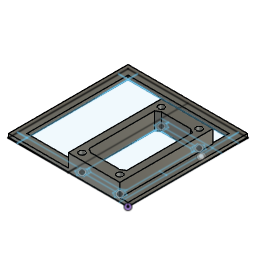
Redstone ESP 8266 Bracket v4 (Autodesk Fusion 360 design; units mm, degrees)
Autodesk Fusion 360 part; units mm, degrees
note: some values were not read from the file. Set by a fixed rule: which sketch regions a step uses.
sketch "Sketch1" plane through (0, 0, 0) normal (0, 0, 1) x (1, 0, 0)
  line L0 (0, 0) -> (-65, 0)
  line L1 (-65, 0) -> (-65, 65)
  line L2 (-65, 65) -> (0, 65)
  line L3 (0, 65) -> (0, 0)
  line L4 (-32.5, 65) -> (-32.5, 0)
  line L5 (-28.75, 1) -> (-26.3684, 2.375)
  line L6 (-26.3684, 2.375) -> (-26.3684, 5.125)
  line L7 (-26.3684, 5.125) -> (-28.75, 6.5)
  line L8 (-28.75, 6.5) -> (-31.1316, 5.125)
  line L9 (-31.1316, 5.125) -> (-31.1316, 2.375)
  line L10 (-31.1316, 2.375) -> (-28.75, 1)
  line L11 (-28.75, 44.19) -> (-26.3684, 45.565)
  line L12 (-26.3684, 45.565) -> (-26.3684, 48.315)
  line L13 (-26.3684, 48.315) -> (-28.75, 49.69)
  line L14 (-28.75, 49.69) -> (-31.1316, 48.315)
  line L15 (-31.1316, 48.315) -> (-31.1316, 45.565)
  line L16 (-31.1316, 45.565) -> (-28.75, 44.19)
  line L17 (-28.75, 49.69) -> (-28.75, 50.69)
  line L18 (-28.75, 50.69) -> (-32.5, 50.69)
  line L19 (-28.75, 50.69) -> (0, 50.69)
  line L20 (-65, 0) -> (-60, 0)
  line L21 (-60, 0) -> (-60, 5)
  line L22 (-60, 5) -> (-65, 5)
  line L23 (-65, 5) -> (-65, 0)
  line L24 (-65, 65) -> (-60, 65)
  line L25 (-60, 65) -> (-60, 60)
  line L26 (-60, 60) -> (-65, 60)
  line L27 (-65, 60) -> (-65, 65)
  line L28 (0, 65) -> (-5, 65)
  line L29 (-5, 65) -> (-5, 60)
  line L30 (-5, 60) -> (0, 60)
  line L31 (0, 60) -> (0, 65)
  line L32 (-5, 60) -> (-60, 60)
  line L33 (-60, 60) -> (-60, 65)
  line L34 (-60, 65) -> (-5, 65)
  line L35 (-5, 65) -> (-5, 60)
  line L36 (-60, 60) -> (-65, 60)
  line L37 (-65, 60) -> (-65, 5)
  line L38 (-65, 5) -> (-60, 5)
  line L39 (-60, 5) -> (-60, 60)
  line L40 (-60, 0) -> (-32.5, 0)
  line L41 (-32.5, 0) -> (-32.5, 5)
  line L42 (-32.5, 5) -> (-60, 5)
  line L43 (-60, 5) -> (-60, 0)
  line L44 (-28.75, 6.5) -> (-28.75, 7.5)
  line L45 (-28.75, 7.5) -> (-26.3684, 6.125)
  line L46 (-28.75, 44.19) -> (-28.75, 43.19)
  line L47 (-3.75, 44.19) -> (-3.75, 43.19)
  line L48 (-26.3684, 44.565) -> (-28.75, 43.19)
  line L49 (-28.75, 7.5) -> (-28.75, 43.19)
  circle A0 centre (-28.75, 46.94) radius 1.65
  circle A1 centre (-28.75, 3.75) radius 1.65
  line L50 (-5, 60) -> (-5, 50.69)
  line L51 (-28.75, 46.94) -> (-8.2, 46.94)
  circle A2 centre (-8.2, 46.94) radius 1.65
  line L52 (-28.75, 3.75) -> (-8.2, 3.75)
  circle A3 centre (-8.2, 3.75) radius 1.65
  line L53 (-8.2, 1) -> (-5.8184, 2.375)
  line L54 (-5.8184, 2.375) -> (-5.8184, 5.125)
  line L55 (-5.8184, 5.125) -> (-8.2, 6.5)
  line L56 (-8.2, 6.5) -> (-10.5816, 5.125)
  line L57 (-10.5816, 5.125) -> (-10.5816, 2.375)
  line L58 (-10.5816, 2.375) -> (-8.2, 1)
  line L59 (-8.2, 44.19) -> (-5.8184, 45.565)
  line L60 (-5.8184, 45.565) -> (-5.8184, 48.315)
  line L61 (-5.8184, 48.315) -> (-8.2, 49.69)
  line L62 (-8.2, 49.69) -> (-10.5816, 48.315)
  line L63 (-10.5816, 48.315) -> (-10.5816, 45.565)
  line L64 (-10.5816, 45.565) -> (-8.2, 44.19)
  line L65 (-8.2, 44.19) -> (-8.2, 43.19)
  line L66 (-8.2, 43.19) -> (-10.5816, 44.565)
  line L67 (-10.5816, 44.565) -> (-26.3684, 44.565)
  line L68 (-8.2, 43.19) -> (-8.2, 7.5)
  line L69 (-8.2, 7.5) -> (-10.5816, 6.125)
  line L70 (-10.5816, 6.125) -> (-26.3684, 6.125)
  line L71 (-8.2, 25.345) -> (-4.45, 25.345)
  line L72 (-4.45, 25.345) -> (-4.45, 0)
  line L73 (-4.45, 25.345) -> (-4.45, 50.69)
  point P0 (-28.75, 3.75)
  point P1 (-28.75, 46.94)
  point P2 (-8.2, 3.75)
  point P3 (-8.2, 46.94)
  dimension "d1" = 65
  dimension "d2" = 65
  dimension "d10" = 43.19
  dimension "d12" = 2.75
  dimension "d14" = 1
  dimension "d15" = 1
  dimension "d17" = 3.3
  dimension "d20" = 3.3
  dimension "d27" = 20.55
  dimension "d28" = 3.3
  dimension "d29" = 20.55
  dimension "d30" = 3.3
  dimension "d31" = 2.75
  dimension "d32" = 1
  dimension "d33" = 3.75
  constraint horizontal L0
  constraint vertical L1
  constraint horizontal L2
  constraint vertical L3
  constraint coincident L0.start L3.end
  constraint midpoint L2 L4.start
  constraint midpoint L0 L4.end
  constraint vertical L17
  constraint coincident L4 L18.end
  constraint perpendicular L4 L18
  constraint coincident L3 L19.end
  constraint perpendicular L3 L19
  constraint horizontal L20
  constraint vertical L21
  constraint horizontal L22
  constraint vertical L23
  constraint horizontal L24
  constraint vertical L25
  constraint horizontal L26
  constraint vertical L27
  constraint horizontal L28
  constraint vertical L29
  constraint horizontal L30
  constraint vertical L31
  constraint horizontal L32
  constraint vertical L33
  constraint horizontal L34
  constraint vertical L35
  constraint horizontal L36
  constraint vertical L37
  constraint horizontal L38
  constraint vertical L39
  constraint horizontal L40
  constraint vertical L41
  constraint horizontal L42
  constraint vertical L43
  constraint coincident L4 L41.end
  constraint vertical L44
  constraint parallel L7 L45
  constraint vertical L46
  constraint perpendicular L19 L47
  constraint parallel L11 L48
  constraint parallel L46 L49
  constraint coincident P1 A0.centre
  constraint coincident P0 A1.centre
  constraint coincident L19 L50.end
  constraint perpendicular L19 L50
  constraint perpendicular L12 L51
  constraint coincident P3 L51.end
  constraint perpendicular L49 L52
  constraint coincident P2 L52.end
  constraint vertical L65
  constraint parallel L64 L66
  constraint horizontal L67
  constraint perpendicular L67 L68
  constraint parallel L56 L69
  constraint parallel L67 L70
  constraint midpoint L68 L71.start
  constraint perpendicular L68 L71
  constraint coincident L0 L72.end
  constraint perpendicular L0 L72
  constraint coincident L19 L73.end
  constraint perpendicular L19 L73
  measures "d1" distance of L0.start L0.end
  measures "d2" distance of L0.start L2.end
  measures "d10" distance of P0 P1
  measures "d12" distance of L11.start P1
  measures "d14" distance of L13.end L17.end
  measures "d15" distance of L11.start L46.end
  measures "d17" diameter of A0
  measures "d20" diameter of A1
  measures "d27" distance of P1 P3
  measures "d28" diameter of A2
  measures "d29" distance of P0 P2
  measures "d30" diameter of A3
  measures "d31" distance of L59.start P3
  measures "d32" distance of L59.start L65.end
  measures "d33" distance of L71.start L71.end
extrude "Extrude4" add sketch "Sketch1" along normal blind 9.2 contours L0 L4 L14 L15 L16 L17 L18 L41 L45 L46 L49 L68 L69 L70 L71 L72 | L12 L13 L17 L19 L51 L59 L60 L61 L62 L63 L65 L68 L71 L73 | L11 L12 L46 L48 L51 L63 L64 L65 L66 L67 | L59 L60 L61 L62 L63 L64 | L11 L12 L13 L14 L15 L16 | L5 L6 L7 L8 L9 L10 | L53 L54 L55 L56 L57 L58
extrude "Extrude5" add sketch "Sketch1" along normal blind 2 contours L0 L3 L19 L72 L73 | L3 L19 L30 L50 | L0 L4 L21 L40 L41 L42 L43 | L2 L3 L28 L29 L30 L31 L35 | L0 L1 L20 L21 L22 L23 L38 L43 | L2 L4 L29 L32 L34 L35 | L1 L22 L26 L36 L37 L38 L39 | L2 L4 L25 L32 L33 L34 | L1 L2 L24 L25 L26 L27 L33 L36
extrude "Extrude6" cut sketch "Sketch1" along normal blind 6 contours L59 L60 L61 L62 L63 L64 | L11 L12 L13 L14 L15 L16 | L5 L6 L7 L8 L9 L10 | L53 L54 L55 L56 L57 L58
